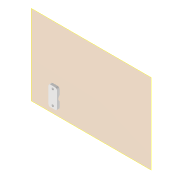
# Autodesk Inventor part: 20_Laserlauncher_Fixation
Saved by Autodesk Inventor 2022 (Build 260153000, 153)
## iProperties
Created: 2022-09-19
Part Number: 20_Laserlauncher_Fixation
Material: Generisch
Document SubType Name: Modeling
Designer: UC2
Density: 1 g/cm^3
Appearance: Vorgabe
Author: UC2
Autodesk Inventor part; units mm, degrees
ref_plane "YZ Plane" through (0, 0, 0) normal (1, 0, 0) x (0, 1, 0)
ref_plane "XZ Plane" through (0, 0, 0) normal (0, 1, 0) x (-1, 0, 0)
ref_plane "XY Plane" through (0, 0, 0) normal (0, 0, 1) x (1, 0, 0)
ref_plane "Arbeitsebene1" through (0, 0, 0) normal (0, 0, 1) x (1, 0, 0)
sketch "Skizze1" plane through (0, 0, 0) normal (0, 0, 1) x (1, 0, 0)
  circle A0 centre (-42.2276, -19.25) radius 1.4 projected
  circle A1 centre (-42.2276, -36.25) radius 1.4 projected
  line L0 (-63.9, -22.9942) -> (-41.36, -22.9942) projected
  line L1 (-41.36, -32.5058) -> (-63.9, -32.5058) projected
  line L2 (-37.2276, -39.25) -> (-47.2276, -39.25)
  line L3 (-47.2276, -39.25) -> (-47.2276, -16.25)
  line L4 (-47.2276, -16.25) -> (-37.2276, -16.25)
  line L5 (-37.2276, -16.25) -> (-37.2276, -39.25)
  line L6 (-37.2276, -39.25) -> (-47.2276, -16.25) construction
  line L7 (-47.2276, -39.25) -> (-37.2276, -16.25) construction
  point P0 (0, 0)
  point P1 (-42.2276, -27.75)
  dimension "d0" = 10
  dimension "d1" = 3
  dimension "d2" = 3
  constraints: 12 end point, 2 midpoint, 2 parallel, 1 horizontal, 1 perpendicular
  measures "d0" distance of L3.end L4.end
  measures "d1" distance from line of A0.centre L4
  measures "d2" distance from line of L2 A1.centre
extrude "Extrusion1" add sketch "Skizze1" along normal blind 3
fillet "Rundung1" radius 2 4 edges at (-37.2276, -16.25, 1.5) (-37.2276, -39.25, 1.5) (-47.2276, -39.25, 1.5) (-47.2276, -16.25, 1.5)
sketch "Skizze2" plane through (-37.2276, -37.25, 0) normal (1, 0, 0) x (0, 0, -1)
  line L0 (0, 13.5) -> (4.8526, 13.5) projected
  circle A0 centre (4.8526, 9.5) radius 7 projected
  circle A1 centre (3.1016, 9.5) radius 4.5
  point P0 (0, 37.25)
  dimension "d6" = 9
  constraints: 1 centre point
  measures "d6" diameter of A1
extrude "Extrusion2" cut sketch "Skizze2" against normal through all contours A1
